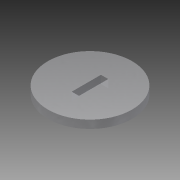
# Autodesk Inventor part: open4
Saved by Autodesk Inventor 2015 (Build 190159000, 159)
## iProperties
Created: 2015-02-17
Part Number: open4
Material: Plastic, Transparent
Document SubType Name: Modeling
Designer: Hanjie
Density: 1.188 g/cm^3
Appearance: Transparent - Clear
Author: Hanjie
Autodesk Inventor part; units mm, degrees
ref_plane "YZ Plane" through (0, 0, 0) normal (1, 0, 0) x (0, 1, 0)
ref_plane "XZ Plane" through (0, 0, 0) normal (0, 1, 0) x (-1, 0, 0)
ref_plane "XY Plane" through (0, 0, 0) normal (0, 0, 1) x (1, 0, 0)
sketch "Sketch1" plane through (0, 0, 0) normal (0, 1, 0) x (-1, 0, 0)
  circle A0 centre (0, 0) radius 29.21
  dimension "d0" = 58.42
  constraints: 1 centre point, 1 coincident
  measures "d0" diameter of A0
extrude "Extrusion1" add sketch "Sketch1" along normal blind 5.588
sketch "Sketch2" plane through (0, 5.588, 0) normal (0, 1, 0) x (1, 0, 0)
  line L0 (0, 0) -> (0, -10.16)
  line L1 (0, -10.16) -> (-2.54, -10.16)
  line L2 (-2.54, -10.16) -> (2.54, -10.16)
  line L3 (2.54, -10.16) -> (2.54, 10.16)
  line L4 (2.54, 10.16) -> (-2.54, 10.16)
  line L5 (-2.54, 10.16) -> (-2.54, -10.16)
  dimension "d3" = 10.16
  dimension "d4" = 2.54
  dimension "d5" = 5.08
  dimension "d6" = 20.32
  constraints: 12 end point, 2 horizontal, 2 parallel, 1 perpendicular, 1 vertical
  measures "d3" distance of L0.start L0.end
  measures "d4" distance of L0.end L1.end
  measures "d5" distance of L4.end L3.end
  measures "d6" distance of L3.end L2.end
extrude "Extrusion2" cut sketch "Sketch2" against normal blind 5.588
body "Solid1"
